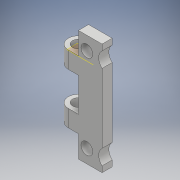
# Autodesk Inventor part: k2_hinge1_bot
Saved by Autodesk Inventor 2017 (Build 210142000, 142)
## iProperties
Created: 2017-02-14
Part Number: k2_hinge1_bot
Material: Generic
Document SubType Name: Modeling
Designer: herman
Density: 1 g/cm^3
Appearance: Default
Author: herman
Autodesk Inventor part; units mm, degrees
ref_plane "YZ Plane" through (0, 0, 0) normal (1, 0, 0) x (0, 1, 0)
ref_plane "XZ Plane" through (0, 0, 0) normal (0, 1, 0) x (-1, 0, 0)
ref_plane "XY Plane" through (0, 0, 0) normal (0, 0, 1) x (1, 0, 0)
sketch "Sketch2" plane through (0, 0, 0) normal (0, 1, 0) x (-1, 0, 0)
  line L0 (8.7236, 13.4517) -> (-1.2764, 13.4517)
  line L1 (-1.2764, 13.4517) -> (-1.2764, -3.0483)
  line L2 (-1.2764, -3.0483) -> (8.7236, -3.0483)
  line L3 (8.7236, -3.0483) -> (8.7236, 13.4517)
  point P0 (0, 0)
  dimension "d2" = 10
  dimension "d3" = 16.5
  constraints: 8 end point, 2 parallel, 1 horizontal, 1 perpendicular
  measures "d2" distance of L2.end L1.end
  measures "d3" distance of L1.end L0.end
extrude "Extrusion1" add sketch "Sketch2" along normal blind 3
ref_plane "Work Plane1" through (-8.7236, 0, 6.9517) normal (0, 0, 1) x (1, 0, 0)
sketch "Sketch5" plane through (-8.7236, 0, 13.4517) normal (0, 0, 1) x (1, 0, 0)
  line L0 (0, 3) -> (10, 3) projected
  line L1 (-3, 0) -> (3, 0)
  line L2 (3, 0) -> (3, 6)
  line L3 (3, 6) -> (-3, 6)
  line L4 (-3, 6) -> (-3, 0)
  line L5 (0, 0) -> (10, 0) projected
  point P0 (8.7236, 0)
  dimension "d41" = 6
  dimension "d42" = 6
  dimension "d43" = 3
  constraints: 8 end point, 2 parallel, 1 horizontal, 1 midpoint, 1 perpendicular, 1 point on line
  measures "d41" distance of L2.end L3.end
  measures "d42" distance of L3.end L1.start
  measures "d43" distance of L5.start L1.end
extrude "Extrusion4" cut sketch "Sketch5" against normal blind 6.5
sketch "Sketch6" plane through (-8.7236, 0, 6.9517) normal (0, 0, 1) x (1, 0, 0)
  circle A0 centre (0, 3) radius 3
  arc A1 (0, 0) -> (3, 3) centre (0, 3) ccw projected
  point P0 (8.7236, 0)
  point P1 (0, 0.5)
  dimension "d16" = 6
  constraints: 1 centre point, 1 coincident, 1 other
  measures "d16" diameter of A0
extrude "Extrusion5" add sketch "Sketch6" against normal blind 5
sketch "Sketch7" plane through (-8.7236, 0, 6.9517) normal (0, 0, 1) x (1, 0, 0)
  arc A0 (3, 3) -> (0, 0) centre (0, 3) ccw projected
  circle A1 centre (0, 3) radius 1.75
  line L0 (3, 0) -> (0, 0) projected
  line L1 (3, 3) -> (3, 0) projected
  point P0 (8.7236, 0)
  dimension "d20" = 3.5
  constraints: 1 centre point, 1 coincident
  measures "d20" diameter of A1
extrude "Extrusion6" cut sketch "Sketch7" against normal up to next contours A1
sketch "Sketch9" plane through (0, 3, 0) normal (0, 1, 0) x (1, 0, 0)
  circle A0 centre (-3.2236, -9.4517) radius 1.75
  line L0 (1.2764, -13.4517) -> (1.2764, 3.0483) projected
  line L1 (-5.7236, -13.4517) -> (1.2764, -13.4517) projected
  point P0 (0, 0)
  dimension "d28" = 3.5
  dimension "d29" = 4.5
  dimension "d30" = 4
  constraints: 1 centre point
  measures "d28" diameter of A0
  measures "d29" distance from line of L0 A0.centre
  measures "d30" distance from line of A0.centre L1
extrude "Extrusion8" cut sketch "Sketch9" against normal up to next
mirror "Mirror2" about plane through (1.2764, 0, -3.0483) normal (0, 0, -1)
sketch "Sketch10" plane through (0, 3, 0) normal (0, 1, 0) x (1, 0, 0)
  circle A0 centre (3.2764, -9.4517) radius 3
  circle A1 centre (3.2764, 15.5483) radius 3
  line L0 (1.2764, -13.4517) -> (1.2764, 19.5483) projected
  point P0 (0, 0)
  dimension "d33" = 6
  dimension "d34" = 6
  dimension "d35" = 2
  dimension "d36" = 4
  dimension "d37" = 4
  dimension "d40" = 2
  constraints: 2 centre point
  measures "d33" diameter of A0
  measures "d34" diameter of A1
  measures "d35" distance from line of L0 A0.centre
  measures "d36" vertical distance of L0.start A0.centre
  measures "d37" vertical distance of L0.end A1.centre
  measures "d40" distance from line of L0 A1.centre
extrude "Extrusion9" cut sketch "Sketch10" against normal through all
sketch "Sketch11" plane through (-8.7236, 0, 1.9517) normal (0, 0, -1) x (-1, 0, 0)
  line L0 (-3, 0) -> (-10, 0) projected
  line L1 (-3, 0) -> (3, 0)
  line L2 (3, 0) -> (3, 6)
  line L3 (3, 6) -> (-3, 6)
  line L4 (-3, 6) -> (-3, 0)
  point P0 (-8.7236, 0)
  dimension "d44" = 6
  dimension "d45" = 6
  constraints: 8 end point, 2 parallel, 1 horizontal, 1 perpendicular
  measures "d44" distance of L0.start L1.end
  measures "d45" distance of L1.end L2.end
extrude "Extrusion10" cut sketch "Sketch11" along normal blind 10
equation "\"d33\" = d34"
equation "\"d37\" = d36"
equation "\"d40\" = d35"
body "Solid1"
